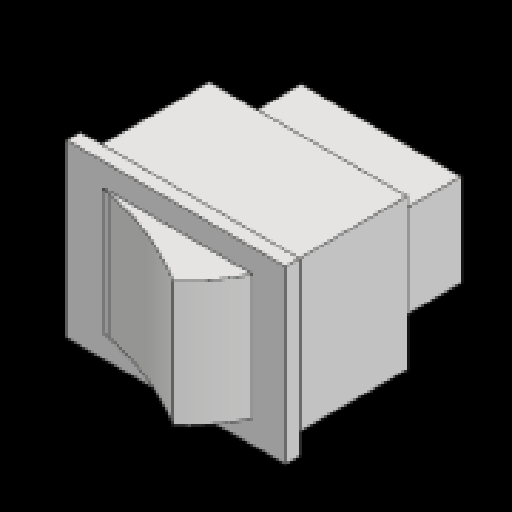
# Autodesk Inventor part: IlluminatedSwitch12V10A
Saved by Autodesk Inventor 2025.2 (Build 292293000, 293)
## iProperties
Created: 2026-06-05
Part Number: IlluminatedSwitch12V10A
Material: Generic
Document SubType Name: Modeling
Designer: valer
Density: 1 g/cm^3
Appearance: Default
Author: valer
Autodesk Inventor part; units mm, degrees
ref_plane "YZ Plane" through (0, 0, 0) normal (1, 0, 0) x (0, 1, 0)
ref_plane "XZ Plane" through (0, 0, 0) normal (0, 1, 0) x (-1, 0, 0)
ref_plane "XY Plane" through (0, 0, 0) normal (0, 0, 1) x (1, 0, 0)
sketch "Base" plane through (0, 0, 0) normal (0, 0, 1) x (1, 0, 0)
  line L0 (-15.748, -12.319) -> (15.748, -12.319)
  line L1 (15.748, -12.319) -> (15.748, 12.319)
  line L2 (15.748, 12.319) -> (-15.748, 12.319)
  line L3 (-15.748, 12.319) -> (-15.748, -12.319)
  line L4 (-15.748, -12.319) -> (15.748, 12.319) construction
  line L5 (15.748, -12.319) -> (-15.748, 12.319) construction
  point P0 (0, 0)
  dimension "d0" = 31.496
  dimension "d1" = 24.638
  constraints: 12 end point, 2 midpoint, 2 parallel, 1 horizontal, 1 perpendicular
  measures "d0" distance of L1.end L2.end
  measures "d1" distance of L2.end L0.start
extrude "BaseFeature" add sketch "Base" along normal blind 2
sketch "Switch" plane through (0, 0, 2) normal (0, 0, 1) x (1, 0, 0)
  line L0 (-12, -9) -> (12, -9)
  line L1 (12, -9) -> (12, 9)
  line L2 (12, 9) -> (-12, 9)
  line L3 (-12, 9) -> (-12, -9)
  line L4 (-12, -9) -> (12, 9) construction
  line L5 (12, -9) -> (-12, 9) construction
  point P0 (0, 0)
  dimension "d4" = 24
  dimension "d7" = 18
  constraints: 12 end point, 2 midpoint, 2 parallel, 1 horizontal, 1 perpendicular
  measures "d4" distance of L0.start L0.end
  measures "d7" distance of L0.end L1.end
extrude "SwitchFeature" add sketch "Switch" along normal blind 6.5
sketch "SwitchProfile" plane through (-12, -9, 2) normal (0, -1, 0) x (1, 0, 0)
  line L0 (27.748, 0) -> (-3.748, 0) projected
  line L1 (24, 6.5) -> (0, 6.5) projected
  arc A0 (23, 0) -> (18, 6.5) centre (5.3894, -8.3735) ccw
  arc A1 (2.5453, 0.2566) -> (18, 6.5) centre (-6.2914, 44.3804) ccw
  arc A2 (2.5453, 0.2566) -> (1.5, 0) centre (5, -12) ccw
  line L2 (24, 0) -> (24, 6.5) projected
  line L3 (0, 0) -> (0, 6.5) projected
  point P0 (12, -2)
  point P1 (0, 3.25)
  dimension "d8" = 6
  dimension "d10" = 45
  dimension "d11" = 19.5
  dimension "d13" = 12.5
  dimension "d14" = 1
  dimension "d15" = 12
  dimension "d16" = 19
  constraints: 6 point on circle, 3 centre point, 3 point on line, 1 midpoint, 1 tangent
  measures "d8" distance from line of L2 A0.end
  measures "d10" radius of A1
  measures "d11" radius of A0
  measures "d13" radius of A2
  measures "d14" distance from line of A0.start L2
  measures "d15" distance from line of A2.centre L0
  measures "d16" distance from line of A2.centre L2
extrude "SwitchProfileFeature" cut sketch "SwitchProfile" against normal through all contours L0 A0 L1 L2 | L0 L3 L1 A1 A2
sketch "Body" plane through (0, 0, 0) normal (0, 0, -1) x (-1, 0, 0)
  line L0 (-14.224, -10.795) -> (14.224, -10.795)
  line L1 (14.224, -10.795) -> (14.224, 10.795)
  line L2 (14.224, 10.795) -> (-14.224, 10.795)
  line L3 (-14.224, 10.795) -> (-14.224, -10.795)
  line L4 (-14.224, -10.795) -> (14.224, 10.795) construction
  line L5 (14.224, -10.795) -> (-14.224, 10.795) construction
  line L6 (15.748, -12.319) -> (-15.748, -12.319) projected
  line L7 (15.748, 12.319) -> (15.748, -12.319) projected
  point P0 (0, 0)
  dimension "d19" = 21.59
  dimension "d20" = 1.524
  dimension "d21" = 1.524
  constraints: 12 end point, 2 midpoint, 2 parallel, 1 horizontal, 1 perpendicular
  measures "d19" distance of L0.end L1.end
  measures "d20" distance between parallel lines of L6 L0
  measures "d21" distance between parallel lines of L7 L1
extrude "BodyFeature" add sketch "Body" along normal blind 17
sketch "Pins" plane through (0, 0, -17) normal (0, 0, -1) x (-1, 0, 0)
  line L0 (11.5, -6.6456) -> (-11.5, -6.6456)
  line L1 (-11.5, -6.6456) -> (-11.5, 6.6456)
  line L2 (-11.5, 6.6456) -> (11.5, 6.6456)
  line L3 (11.5, 6.6456) -> (11.5, -6.6456)
  line L4 (11.5, -6.6456) -> (-11.5, 6.6456) construction
  line L5 (-11.5, -6.6456) -> (11.5, 6.6456) construction
  line L6 (-14.224, -10.795) -> (14.224, -10.795) projected
  point P0 (0, 0)
  point P1 (0, -10.795)
  dimension "d25" = 23
  constraints: 12 end point, 3 midpoint, 2 parallel, 1 horizontal, 1 perpendicular
  measures "d25" distance between parallel lines of L1 L3
extrude "PinsFeature" add sketch "Pins" along normal blind 10.5
equation "\"d21\" = d20"
body "Solid1"
